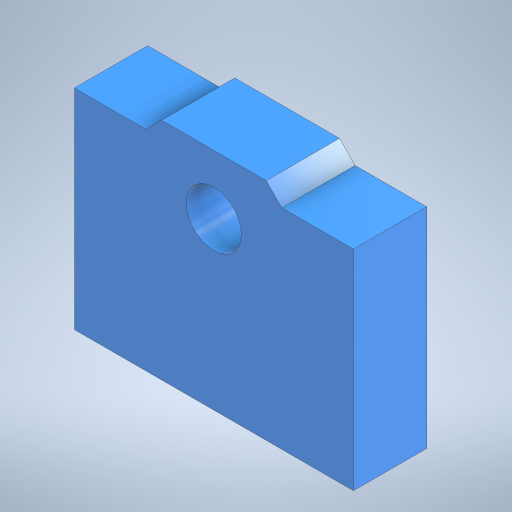
# Autodesk Inventor part: Roller Bracket
Saved by Autodesk Inventor 2024 (Build 280153020, 153B)
## iProperties
Created: 2024-02-06
Part Number: Roller Bracket
Material: Generic
Document SubType Name: Modeling
Designer: scottst
Density: 1 g/cm^3
Appearance: Default
Author: scottst
Autodesk Inventor part; units mm, degrees
sketch "Sketch3" plane through (0, 0, 0) normal (0, 1, 0) x (-1, 0, 0)
  line L0 (-20.32, 6.35) -> (20.32, 6.35)
  line L1 (20.32, 6.35) -> (20.32, -6.35)
  line L2 (20.32, -6.35) -> (-20.32, -6.35)
  line L3 (-20.32, -6.35) -> (-20.32, 6.35)
  line L4 (-20.32, 6.35) -> (20.32, -6.35) construction
  line L5 (20.32, 6.35) -> (-20.32, -6.35) construction
  point P0 (0, 0)
  dimension "d0" = 40.64
  dimension "d1" = 12.7
  constraints: 12 end point, 2 midpoint, 2 parallel, 1 horizontal, 1 perpendicular
  measures "d0" distance of L1.end L2.end
  measures "d1" distance of L0.end L1.end
sketch "Sketch3 outline for Extrusion1" plane through (0, 0, 0) normal (0, 1, 0) x (-1, 0, 0)
  line L0 (-20.32, 6.35) -> (-20.32, -6.35)
  line L1 (20.32, 6.35) -> (-20.32, 6.35)
  line L2 (20.32, -6.35) -> (20.32, 6.35)
  line L3 (-20.32, -6.35) -> (20.32, -6.35)
extrude "Extrusion1" add sketch "Sketch3 outline for Extrusion1" along normal blind 30.48
sketch "Sketch4" plane through (-20.32, 0, 6.35) normal (0, 0, 1) x (1, 0, 0)
  line L0 (20.32, 0) -> (20.32, 24.13) construction
  circle A0 centre (20.32, 24.13) radius 4
  line L1 (12.7, 28.196818) -> (27.94, 28.196818)
  line L2 (27.94, 28.196818) -> (27.94, 32.763182)
  line L3 (27.94, 32.763182) -> (12.7, 32.763182)
  line L4 (12.7, 32.763182) -> (12.7, 28.196818)
  line L5 (40.64, 30.48) -> (0, 30.48)
  line L6 (12.7, 28.196818) -> (27.94, 32.763182) construction
  line L7 (27.94, 28.196818) -> (12.7, 32.763182) construction
  point P0 (20.32, 30.48)
  dimension "d4" = 24.13
  dimension "d5" = 8
  dimension "d6" = 15.24
  constraints: 14 end point, 3 midpoint, 2 parallel, 1 centre point, 1 coincident, 1 horizontal, 1 perpendicular, 1 vertical
  measures "d4" distance of L0.start L0.end
  measures "d5" diameter of A0
  measures "d6" distance of L3.end L2.end
sketch "Sketch4 outline for Extrusion2" plane through (-20.32, 0, 6.35) normal (0, 0, 1) x (1, 0, 0)
  line L0 (27.94, 32.763182) -> (12.7, 32.763182)
  line L1 (27.94, 28.196818) -> (27.94, 32.763182)
  line L2 (12.7, 28.196818) -> (27.94, 28.196818)
  line L3 (12.7, 32.763182) -> (12.7, 28.196818)
extrude "Extrusion2" add sketch "Sketch4 outline for Extrusion2" against normal up to surface (12.7 mm away)
sketch "Sketch4 outline for Extrusion3" plane through (-20.32, 0, 6.35) normal (0, 0, 1) x (1, 0, 0)
  circle A0 centre (20.32, 24.13) radius 4
extrude "Extrusion3" cut sketch "Sketch4 outline for Extrusion3" against normal blind 22.225
chamfer "Chamfer1" distance 2.28092 angle 45 2 edges at (7.62, 30.48, 0) (-7.62, 30.48, 0)
sketch "Sketch5" plane through (0, 0, 0) normal (0, -1, 0) x (1, 0, 0)
  line L0 (0, 0) -> (-12.7, 0) construction
  line L1 (0, 0) -> (12.7, 0) construction
  circle A0 centre (-12.7, 0) radius 1.65
  circle A1 centre (12.7, 0) radius 1.65
  dimension "d14" = 12.7
  dimension "d15" = 12.7
  dimension "d16" = 3.3
  dimension "d17" = 3.3
  constraints: 4 end point, 2 centre point, 2 coincident, 2 horizontal
  measures "d14" distance of L0.start L0.end
  measures "d15" distance of L0.start L1.end
  measures "d16" diameter of A0
  measures "d17" diameter of A1
sketch "Sketch5 outline for Extrusion4" plane through (0, 0, 0) normal (0, -1, 0) x (1, 0, 0)
  circle A0 centre (12.7, 0) radius 1.65
  circle A1 centre (-12.7, 0) radius 1.65
extrude "Extrusion4" cut sketch "Sketch5 outline for Extrusion4" against normal blind 20
ref_plane "Work Plane1" through (20.32, 0, -4.318) normal (0, 0, -1) x (-1, 0, 0)
sketch "Sketch6" plane through (20.32, 0, -4.318) normal (0, 0, -1) x (-1, 0, 0)
  line L0 (0, 30.48) -> (10.41908, 30.48)
  line L1 (0, 0) -> (0, 30.48)
  line L2 (0, 0) -> (40.64, 0)
  line L3 (40.64, 0) -> (40.64, 30.48)
  line L4 (30.22092, 30.48) -> (40.64, 30.48)
  line L5 (27.94, 32.76092) -> (30.22092, 30.48)
  line L6 (12.7, 32.763182) -> (27.94, 32.763182)
  line L7 (10.41908, 30.48) -> (12.7, 32.76092)
  circle A0 centre (20.32, 24.13) radius 4
  line L8 (0, 30.48) -> (10.41908, 30.48)
  line L9 (0, 0) -> (0, 30.48)
  line L10 (0, 0) -> (40.64, 0)
  line L11 (40.64, 0) -> (40.64, 30.48)
  line L12 (30.22092, 30.48) -> (40.64, 30.48)
  line L13 (27.94, 32.76092) -> (30.22092, 30.48)
  line L14 (27.94, 32.763182) -> (27.94, 32.76092)
  line L15 (12.7, 32.763182) -> (27.94, 32.763182)
  line L16 (12.7, 32.76092) -> (12.7, 32.763182)
  line L17 (10.41908, 30.48) -> (12.7, 32.76092)
  line L18 (0, 30.48) -> (0, 0)
  line L19 (40.64, 0) -> (0, 0)
  line L20 (40.64, 0) -> (40.64, 30.48)
  line L21 (40.64, 30.48) -> (30.22092, 30.48)
  line L22 (30.22092, 30.48) -> (27.94, 32.763182)
  line L23 (27.94, 32.763182) -> (12.7, 32.76092)
  line L24 (12.7, 32.76092) -> (10.41908, 30.48)
  line L25 (0, 30.48) -> (10.41908, 30.48)
  point P0 (20.32, 0)
  constraints: 16 end point, 4 perpendicular
sketch "Sketch6 outline for Extrusion5" plane through (20.32, 0, -4.318) normal (0, 0, -1) x (-1, 0, 0)
  line L0 (27.94, 32.76092) -> (27.94, 32.763182)
  line L1 (30.22092, 30.48) -> (27.94, 32.76092)
  line L2 (27.94, 32.763182) -> (12.7, 32.76092)
  line L3 (40.64, 30.48) -> (30.22092, 30.48)
  line L4 (12.7, 32.76092) -> (10.41908, 30.48)
  line L5 (40.64, 0) -> (40.64, 30.48)
  line L6 (10.41908, 30.48) -> (0, 30.48)
  line L7 (0, 0) -> (40.64, 0)
  line L8 (0, 30.48) -> (0, 0)
  circle A0 centre (20.32, 24.13) radius 4
extrude "Extrusion5" cut sketch "Sketch6 outline for Extrusion5" along normal blind 20
sketch "Sketch7" plane through (20.32, 0, -4.318) normal (0, 0, -1) x (-1, 0, 0)
  circle A0 centre (20.32, 24.13) radius 8.255
  point P0 (20.32, 0)
  constraints: 1 centre point
ref_plane "Work Plane2" through (20.32, 0, -5.9055) normal (0, 0, -1) x (-1, 0, 0)
sketch "Sketch8" plane through (20.32, 0, -5.9055) normal (0, 0, -1) x (-1, 0, 0)
  circle A0 centre (20.32, 24.13) radius 5.5
  point P0 (20.32, 0)
  dimension "d25" = 11
  constraints: 1 centre point, 1 coincident
  measures "d25" diameter of A0
sketch "Sketch7 outline for Loft1" plane through (20.32, 0, -4.318) normal (0, 0, -1) x (-1, 0, 0)
  circle A0 centre (20.32, 24.13) radius 8.255
sketch "Sketch8 outline for Loft1" plane through (20.32, 0, -5.9055) normal (0, 0, -1) x (-1, 0, 0)
  circle A0 centre (20.32, 24.13) radius 5.5
loft "Loft1" add profiles "Sketch7 outline for Loft1", "Sketch8 outline for Loft1"
sketch "Sketch9" plane through (-20.32, 0, 6.35) normal (0, 0, 1) x (1, 0, 0)
  circle A0 centre (20.32, 24.13) radius 4 projected
  point P0 (20.32, 0)
sketch "Sketch9 outline for Extrusion6" plane through (-20.32, 0, 6.35) normal (0, 0, 1) x (1, 0, 0)
  circle A0 centre (20.32, 24.13) radius 4
extrude "Extrusion6" cut sketch "Sketch9 outline for Extrusion6" against normal blind 129.224999
ref_plane "Work Plane3" through (0, 10.16, 0) normal (0, -1, 0) x (1, 0, 0)
sketch "Sketch10" plane through (0, 10.16, 0) normal (0, -1, 0) x (1, 0, 0)
  circle A0 centre (-12.7, 0) radius 1.65
  line L0 (-15.5782, 0) -> (-9.87364, 0) construction
  line L1 (-9.90092, 1.631015) -> (-9.90092, -1.631015)
  line L2 (-15.55092, -1.631015) -> (-15.55092, 1.631015)
  line L3 (-12.72592, 3.262029) -> (-9.90092, 1.631015)
  line L4 (-15.55092, 1.631015) -> (-12.72592, 3.262029)
  line L5 (-12.72592, 0) -> (-9.90092, 0) construction
  line L6 (9.84772, 0) -> (15.55228, 0) construction
  line L7 (15.525, 1.631015) -> (15.525, -1.631015)
  line L8 (9.875, -1.631015) -> (9.875, 1.631015)
  line L9 (12.7, 3.262029) -> (15.525, 1.631015)
  line L10 (9.875, 1.631015) -> (12.7, 3.262029)
  line L11 (12.7, 0) -> (15.525, 0) construction
  circle A1 centre (12.7, 0) radius 1.65
  line L12 (15.525, -1.631015) -> (15.525, -3.262029)
  line L13 (15.525, -3.262029) -> (9.875, -3.262029)
  line L14 (9.875, -3.262029) -> (9.875, -1.631015)
  line L15 (-9.90092, -1.631015) -> (-9.90092, -3.262029)
  line L16 (-9.90092, -4.318) -> (-9.90092, 6.35)
  line L17 (-12.72592, -3.262029) -> (-9.90092, -3.262029)
  line L18 (-12.72592, -3.262029) -> (-15.55092, -3.262029)
  line L19 (-15.55092, -3.262029) -> (-15.55092, -1.631015)
  point P0 (0, 0)
  point P1 (-12.7, -1.132545)
  point P2 (-12.7, -3.5)
  point P3 (12.7, -1.132545)
  point P4 (12.7, -3.5)
  dimension "d34" = 2.825
  dimension "d35" = 2.825
  constraints: 38 end point, 4 midpoint, 4 perpendicular, 4 point on line, 2 coincident, 1 vertical, 18 other
  measures "d34" distance of L5.start L5.end
  measures "d35" distance of L11.start L11.end
sketch "Sketch10 outline for Extrusion7" plane through (0, 10.16, 0) normal (0, -1, 0) x (1, 0, 0)
  line L0 (-15.55092, -3.262029) -> (-9.90092, -3.262029)
  line L1 (-9.90092, -3.262029) -> (-9.90092, 1.631015)
  line L2 (-9.90092, 1.631015) -> (-12.72592, 3.262029)
  line L3 (-12.72592, 3.262029) -> (-15.55092, 1.631015)
  line L4 (-15.55092, 1.631015) -> (-15.55092, -3.262029)
  line L5 (15.525, 1.631015) -> (12.7, 3.262029)
  line L6 (12.7, 3.262029) -> (9.875, 1.631015)
  line L7 (9.875, 1.631015) -> (9.875, -3.262029)
  line L8 (9.875, -3.262029) -> (15.525, -3.262029)
  line L9 (15.525, -3.262029) -> (15.525, 1.631015)
extrude "Extrusion7" cut sketch "Sketch10 outline for Extrusion7" along normal mid plane 2.75
sketch "Sketch11" plane through (20.32, 0, -4.318) normal (0, 0, -1) x (-1, 0, 0)
  line L0 (29.08046, 32.526826) -> (11.260311, 32.526826)
  line L1 (11.260311, 32.526826) -> (11.260311, 35.082572)
  line L2 (11.260311, 35.082572) -> (29.08046, 35.082572)
  line L3 (29.08046, 35.082572) -> (29.08046, 32.526826)
  point P0 (20.32, 0)
  constraints: 8 end point, 2 parallel, 1 horizontal, 1 perpendicular
sketch "Sketch11 outline for Extrusion8" plane through (20.32, 0, -4.318) normal (0, 0, -1) x (-1, 0, 0)
  line L0 (29.08046, 32.526826) -> (29.08046, 35.082572)
  line L1 (11.260311, 32.526826) -> (29.08046, 32.526826)
  line L2 (11.260311, 35.082572) -> (11.260311, 32.526826)
  line L3 (29.08046, 35.082572) -> (11.260311, 35.082572)
extrude "Extrusion8" cut sketch "Sketch11 outline for Extrusion8" along normal blind 9.949993
body "Solid1"
